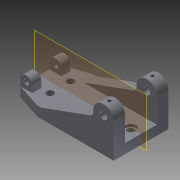
# Autodesk Inventor part: TU-007
Saved by Autodesk Inventor 2011 (Build 150229000, 229)
## iProperties
Created: 2008-07-06
Part Number: TU-007
Document SubType Name: Modeling
Designer: PN
Density: 7.75 g/cm^3
Material: Stainless Steel, 440C
Description: Cylinder Base
Mass: 2332.18 g
Surface Area: 522.777 cm^2
Volume: 300.927 cm^3
Author: PN
Autodesk Inventor part; units mm, degrees
note: some values were not read from the file. Chosen so that the rebuilt part matches the saved one: direction of "Hole3".
ref_plane "YZ Plane" through (0, 0, 0) normal (1, 0, 0) x (0, 1, 0)
sketch "Sketch1" plane through (0, 0, 0) normal (0, 0, 1) x (1, 0, 0)
  line L0 (0, 0) -> (-160, 0)
  line L1 (-160, 0) -> (-160, 86)
  line L2 (-160, 86) -> (0, 86)
  line L3 (0, 86) -> (0, 0)
  dimension "d0" = 160
  dimension "d1" = 86
  constraints: 8 end point, 2 parallel, 1 horizontal, 1 perpendicular
  measures "d0" distance of L0.start L0.end
  measures "d1" distance of L2.end L0.start
extrude "Extrusion1" add sketch "Sketch1" along normal blind 15
sketch "Sketch2" plane through (-160, 0, 0) normal (0, -1, 0) x (1, 0, 0)
  line L0 (160, 15) -> (0, 15) projected
  line L1 (160, 0) -> (0, 0) projected
  line L2 (160, 0) -> (160, 15) projected
  line L3 (160, 15) -> (160, 53)
  arc A0 (160, 53) -> (128, 53) centre (144, 53) ccw
  line L4 (128, 53) -> (128, 45)
  line L5 (128, 45) -> (45.5757, 15)
  dimension "d4" = 16
  dimension "d5" = 53
  dimension "d6" = 20
  dimension "d7" = 8
  constraints: 6 end point, 2 point on circle, 2 tangent, 1 centre point, 1 collinear, 1 parallel, 1 point on line
  measures "d4" radius of A0
  measures "d5" distance from line of A0.centre L1
  measures "d6" angle of L0 L5
  measures "d7" distance of L4.start L4.end
extrude "Extrusion2" add sketch "Sketch2" against normal blind 18
fillet "Fillet1" radius 8 1 edges at (-32, 9, 45)
hole "Hole1" at (-16, 0, 53) direction (0, 1, 0) diameter 11 end through all
ref_plane "Work Plane1" through (-160, 43, 0) normal (0, -1, 0) x (1, 0, 0)
mirror "Mirror1" about plane through (-160, 43, 0) normal (0, -1, 0) of "Extrusion2", "Hole1", "Fillet1"
ref_plane "Work Plane2" through (-160, 13, 0) normal (0, -1, 0) x (1, 0, 0)
sketch "Sketch3" plane through (-160, 13, 0) normal (0, -1, 0) x (1, 0, 0)
  line L0 (45.5757, 15) -> (0, 15) projected
  line L1 (0, 15) -> (0, 25)
  arc A0 (19, 25) -> (0, 25) centre (9.5, 25) ccw
  line L2 (19, 25) -> (19, 15)
  line L3 (160, 0) -> (0, 0) projected
  dimension "d21" = 9.5
  dimension "d22" = 25
  constraints: 4 end point, 2 perpendicular, 2 point on circle, 2 tangent, 1 centre point, 1 point on line
  measures "d21" radius of A0
  measures "d22" distance from line of A0.centre L3
extrude "Extrusion3" add sketch "Sketch3" against normal blind 14
hole "Hole2" at (-150.5, 13, 25) direction (0, 1, 0) diameter 8 end through all
mirror "Mirror2" about plane through (-160, 43, 0) normal (0, -1, 0) of "Extrusion3", "Hole2"
chamfer "Chamfer1" distance 13 distance2 40 1 edges at (-160, 0, 7.5) measured on face at (-160, 37.6667, 5)
chamfer "Chamfer2" distance 13 distance2 40 1 edges at (-160, 86, 7.5) measured on face at (-160, 52.6667, 5)
ref_plane "Work Plane3" through (-16, 0, 69) normal (0, 0, 1) x (1, 0, 0)
sketch "Sketch4" plane through (-16, 0, 69) normal (0, 0, 1) x (1, 0, 0)
  line L0 (-16, 18) -> (16, 18) projected
  line L1 (-16, 0) -> (16, 0) projected
  line L2 (-16, 68) -> (16, 68) projected
  line L3 (-16, 86) -> (16, 86) projected
  line L4 (0, 86) -> (0, 68)
  line L5 (0, 18) -> (0, 0)
  point P0 (0, 77)
  point P1 (0, 9)
  constraints: 6 midpoint, 4 end point
hole "Hole3" at (-16, 77, 69) at (-16, 9, 69) direction (0, 0, -1) diameter 4.917 end up to surface thread size "M6x1" class "6H" standard "ANSI Metric M Profile"
sketch "Sketch5" plane through (0, 0, 15) normal (0, 0, 1) x (1, 0, 0)
  line L0 (-160, 27) -> (-160, 59) projected
  line L1 (32, 43) -> (-192, 43) projected
  point P0 (0, 0)
  point P1 (-127, 59)
  point P2 (-127, 27)
  dimension "d47" = 16
  dimension "d48" = 32
  dimension "d49" = 33
  constraints: 1 vertical alignment
  measures "d47" distance from line of point (-127, 59) L1
  measures "d48" distance of point (-127, 27) point (-127, 59)
  measures "d49" distance from line of point (-127, 27) L0
hole "Hole4" at (-127, 59, 15) at (-127, 27, 15) direction (0, 0, -1) diameter 11 end through all
sketch "Sketch6" plane through (0, 0, 15) normal (0, 0, 1) x (1, 0, 0)
  line L0 (0, 68) -> (0, 18) projected
  line L1 (-120, 86) -> (-114.4243, 86) projected
  line L2 (0, 43) -> (-16, 43)
  point P0 (0, 0)
  dimension "d57" = 16
  constraints: 2 end point, 1 midpoint, 1 parallel
  measures "d57" distance of L2.start L2.end
hole "Hole5" at (-16, 43, 15) direction (0, 0, -1) diameter 11 end through all counterbore diameter 16 counterbore depth 4
equation "\"d48\" = 2 * d47"
body "Solid1"
